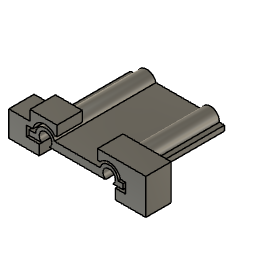
shoe and attachment v0 design (Autodesk Fusion 360 design; units mm, degrees)
Autodesk Fusion 360 part; units mm, degrees
sketch "Sketch1" plane through (0, 0, 0) normal (0, 1, 0) x (1, 0, 0)
  line L0 (-80, -30) -> (100, -30)
  circle A0 centre (-114.9902, -19.7639) radius 25.0021
  circle A1 centre (135.6359, -19.403) radius 24.3858
  line L1 (-260.2482, 49.781) -> (-259.9022, -50.3969)
  line L2 (-259.9022, -50.3969) -> (-176.3717, -50.1084)
  line L3 (-176.3717, -50.1084) -> (-176.2328, -90.3254)
  line L4 (-176.2328, -90.3254) -> (-69.8506, -89.958)
  line L5 (-69.8506, -89.958) -> (-69.9887, -49.9654)
  line L6 (-69.9887, -49.9654) -> (-80, -50)
  line L7 (90, -50) -> (90, -90)
  line L8 (90, -90) -> (280, -90)
  line L9 (280, -90) -> (280, 50)
  line L10 (90, -50) -> (100, -50)
  arc A2 (-154.2538, -19.0176) -> (-80, -30) centre (-116.3853, -19.4949) ccw
  arc A3 (-164.3965, -30) -> (-80, -50) centre (-117.9562, -22.0992) ccw
  line L11 (-154.2538, -19.0176) -> (-176.3829, -19.0176)
  line L12 (-180, -0.0944) -> (-180, -19.0176)
  line L13 (-180, -19.0176) -> (-176.3829, -19.0176)
  line L14 (-180, -0.0944) -> (-130.4244, -0.0944)
  line L15 (121.1929, 0.2455) -> (-99.9993, 0.2455)
  arc A4 (100, -30) -> (170, -20) centre (134.5149, -21.6041) ccw
  arc A5 (100, -50) -> (180, -30) centre (135, -20) ccw
  line L16 (-164.3965, -30) -> (-189.9198, -30.0882)
  line L17 (-189.9198, -30.0882) -> (-190.0573, 9.7235)
  line L18 (-190.0573, 9.7235) -> (-139.9655, 9.8965)
  line L19 (-139.9655, 9.8965) -> (-140.1039, 49.9756)
  line L20 (-140.1039, 49.9756) -> (-260.2474, 49.5606)
  line L21 (150.4071, 0) -> (190.4071, 0)
  line L22 (170, -20) -> (190, -20)
  line L23 (190, -20) -> (190.4071, 0)
  line L24 (180, -30) -> (200, -30)
  line L25 (200, -30) -> (200, 10)
  line L26 (200, 10) -> (160, 10)
  line L27 (160, 10) -> (160, 50)
  line L28 (160, 50) -> (280, 50)
  constraint horizontal L0
  constraint perpendicular L1 L2
  constraint perpendicular L2 L3
  constraint perpendicular L3 L4
  constraint perpendicular L4 L5
  constraint perpendicular L5 L6
  constraint vertical L7
  constraint perpendicular L7 L8
  constraint perpendicular L8 L9
  constraint perpendicular L7 L10
  constraint horizontal L11
  constraint vertical L12
  constraint perpendicular L12 L13
  constraint coincident A0 L14.end
  constraint perpendicular L12 L14
  constraint coincident A1 L15.start
  constraint coincident A0 L15.end
  constraint parallel L14 L15
  constraint parallel L2 L16
  constraint perpendicular L16 L17
  constraint perpendicular L17 L18
  constraint perpendicular L18 L19
  constraint coincident L1 L20.end
  constraint perpendicular L1 L20
  constraint coincident A1 L21.start
  constraint horizontal L21
  constraint parallel L0 L22
  constraint horizontal L24
  constraint perpendicular L24 L25
  constraint perpendicular L25 L26
  constraint perpendicular L26 L27
  constraint coincident L9 L28.end
  constraint perpendicular L9 L28
extrude "Extrude1" add sketch "Sketch1" along normal blind 100 contours L0 A0 A1 A2 L11 L12 L13 L14 L15 A4 L21 L22 L23 | L1 L2 L3 L4 L5 L6 A3 L16 L17 L18 L19 L20 | L7 L8 L9 L10 A5 L24 L25 L26 L27 L28 makes body 1 at (-236.7356, 0, -2.9624) makes body 2 at (47.4622, 33.3333, -0.2455) makes body 3 at (153.3333, 33.3333, 90)
extrude "Extrude2" add 1 faces at (40.4235, 100, 15.2743) along direction (0, 1, 0) blind 300 on bodies 2 bodies 2
